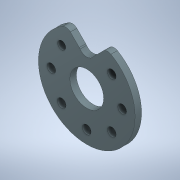
# Autodesk Inventor part: Pulley_middle
Saved by Autodesk Inventor 2020 (Build 240168000, 168)
## iProperties
Created: 2019-10-12
Part Number: Pulley_middle
Material: Generic
Document SubType Name: Modeling
Designer: ayad493
Density: 1 g/cm^3
Appearance: Lead
Author: ayad493
Autodesk Inventor part; units mm, degrees
ref_plane "YZ Plane" through (0, 0, 0) normal (1, 0, 0) x (0, 1, 0)
ref_plane "XZ Plane" through (0, 0, 0) normal (0, 1, 0) x (-1, 0, 0)
ref_plane "XY Plane" through (0, 0, 0) normal (0, 0, 1) x (1, 0, 0)
sketch "Sketch1" plane through (0, 0, 0) normal (0, 0, 1) x (1, 0, 0)
  circle A0 centre (0, 0) radius 18
  dimension "d0" = 36
  constraints: 1 centre point, 1 coincident
  measures "d0" diameter of A0
extrude "Extrusion1" add sketch "Sketch1" along normal blind 2.5
sketch "Sketch2" plane through (0, 0, 2.5) normal (0, 0, 1) x (1, 0, 0)
  line L0 (0, 0) -> (0, 11)
  circle A0 centre (0, 11) radius 1.25
  circle A1 centre (0, 0) radius 5
  circle A2 centre (7.7782, 7.7782) radius 1.25
  circle A3 centre (11, 0) radius 1.25
  circle A4 centre (7.7782, -7.7782) radius 1.25
  circle A5 centre (0, -11) radius 1.25
  circle A6 centre (-7.7782, -7.7782) radius 1.25
  circle A7 centre (-11, 0) radius 1.25
  circle A8 centre (-7.7782, 7.7782) radius 1.25
  dimension "d3" = 11
  dimension "d4" = 2.5
  dimension "d5" = 10
  dimension "d8" = 360
  constraints: 9 centre point, 2 coincident, 2 end point, 1 vertical, 17 other
  measures "d3" distance of L0.start L0.end
  measures "d4" diameter of A0
  measures "d5" diameter of A1
extrude "Extrusion2" cut sketch "Sketch2" against normal through all
sketch "Sketch3" plane through (0, 0, 2.5) normal (0, 0, 1) x (1, 0, 0)
  circle A0 centre (0, 0) radius 15
  circle A1 centre (0, 0) radius 18
  dimension "d12" = 30
  constraints: 2 centre point, 2 coincident
  measures "d12" diameter of A0
extrude "Extrusion3" cut sketch "Sketch3" against normal through all
sketch "Sketch4" plane through (0, 0, 2.5) normal (0, 0, 1) x (1, 0, 0)
  circle A0 centre (0, 11) radius 1.25 projected
  arc A1 (-2.1651, 9.75) -> (2.1651, 9.75) centre (0, 11) ccw
  circle A2 centre (-7.7782, 7.7782) radius 1.25 projected
  circle A3 centre (7.7782, 7.7782) radius 1.25 projected
  circle A4 centre (0, 0) radius 5 projected
  line L0 (2.1651, 9.75) -> (6.1129, 13.6979)
  circle A5 centre (0, 0) radius 15 projected
  line L1 (2.1651, 9.75) -> (7.7482, 9.75) construction
  line L2 (-2.1651, 9.75) -> (-6.1129, 13.6979)
  line L3 (-2.1651, 9.75) -> (3.4181, 9.75) construction
  arc A6 (6.1129, 13.6979) -> (-6.1129, 13.6979) centre (0, 0) ccw
  dimension "d15" = 5
  dimension "d17" = 45
  dimension "d18" = 135
  constraints: 8 end point, 6 point on circle, 2 centre point, 2 equal length, 2 horizontal, 1 coincident, 1 concentric, 1 point on line
  measures "d15" diameter of A1
  measures "d17" angle of L1 L0
  measures "d18" angle of L3 L2
extrude "Extrusion4" cut sketch "Sketch4" against normal blind 10 contours L2 A5 L0 A1 picked at (3.4839, 13.2226)
fillet "Fillet1" radius 2 4 edges at (-6.1129, 13.6979, 1.25) (6.1129, 13.6979, 1.25) (-2.1651, 9.75, 1.25) (2.1651, 9.75, 1.25)
sketch "Sketch5" plane through (0, 0, 2.5) normal (0, 0, 1) x (1, 0, 0)
  line L0 (0, 0) -> (1, 0)
  line L1 (1, 0) -> (1, 1)
  line L2 (1, 1) -> (0, 1)
  line L3 (0, 1) -> (0, 0)
  dimension "d22" = 1
  dimension "d23" = 1
  constraints: 8 end point, 2 parallel, 1 horizontal, 1 perpendicular
  measures "d22" distance of L2.end L1.end
  measures "d23" distance of L1.end L0.end
extrude "Extrusion5" add sketch "Sketch5" along normal blind 1
sketch "Sketch6" plane through (0, 1, 2.5) normal (0, 1, 0) x (1, 0, 0)
  line L0 (2.0766, 0) -> (-2.0766, 0) projected
  line L1 (-15, 2.5) -> (-15, 0) projected
  line L2 (0, 0) -> (-15, 0)
  line L3 (-15, 0) -> (-15, 0.5)
  line L4 (-15, 0.5) -> (0, 0.5)
  line L5 (0, 0.5) -> (0, 0)
  line L6 (0, 0) -> (15, 0)
  line L7 (15, 0) -> (15, 0.5)
  line L8 (15, 0.5) -> (0, 0.5)
  line L9 (0, 0.5) -> (0, 0)
  point P0 (0, 2.5)
  point P1 (0, 0.5)
  dimension "d26" = 0.5
  dimension "d27" = 15
  constraints: 16 end point, 4 parallel, 2 horizontal, 2 perpendicular, 1 midpoint, 1 point on line
  measures "d26" distance of L2.end L3.end
  measures "d27" distance of L8.end L7.end
extrude "Extrusion6" cut sketch "Sketch6" along normal through all both and the other way through all
sketch "Sketch7" plane through (0, 0, 3.5) normal (0, 0, 1) x (1, 0, 0)
  line L0 (1, 1) -> (0, 1) projected
  line L1 (0, 0) -> (1, 0) projected
  line L2 (0, 1) -> (1, 1)
  line L3 (1, 1) -> (1, 0)
  line L4 (1, 0) -> (0, 0)
  line L5 (0, 0) -> (0, 1)
  constraints: 8 end point, 2 parallel, 1 horizontal, 1 perpendicular
extrude "Extrusion7" cut sketch "Sketch7" against normal blind 1
sketch "Sketch8" plane through (0, 0, 2) normal (0, 0, 1) x (1, 0, 0)
  circle A0 centre (0, 0) radius 5.25
  dimension "d32" = 10.5
  constraints: 1 centre point, 1 coincident
  measures "d32" diameter of A0
extrude "Extrusion8" cut sketch "Sketch8" against normal through all
sketch "Sketch9" plane through (0, 0, 0) normal (0, 0, -1) x (-1, 0, 0)
  circle A0 centre (0, -11) radius 1.25 projected
  circle A1 centre (0, -11) radius 1.35
  circle A2 centre (-7.7782, -7.7782) radius 1.25 projected
  circle A3 centre (-7.7782, -7.7782) radius 1.35
  circle A4 centre (-11, 0) radius 1.25 projected
  circle A5 centre (-11, 0) radius 1.35
  circle A6 centre (-7.7782, 7.7782) radius 1.25 projected
  circle A7 centre (-7.7782, 7.7782) radius 1.35
  circle A8 centre (7.7782, -7.7782) radius 1.25 projected
  circle A9 centre (7.7782, -7.7782) radius 1.35
  circle A10 centre (11, 0) radius 1.25 projected
  circle A11 centre (11, 0) radius 1.35
  circle A12 centre (7.7782, 7.7782) radius 1.25 projected
  circle A13 centre (7.7782, 7.7782) radius 1.35
  point P0 (0, 0)
  dimension "d35" = 2.7
  dimension "d36" = 2.7
  dimension "d37" = 2.7
  dimension "d38" = 2.7
  dimension "d39" = 2.7
  dimension "d40" = 2.7
  dimension "d41" = 2.7
  constraints: 7 centre point, 7 coincident
  measures "d35" diameter of A1
  measures "d36" diameter of A3
  measures "d37" diameter of A5
  measures "d38" diameter of A7
  measures "d39" diameter of A9
  measures "d40" diameter of A11
  measures "d41" diameter of A13
extrude "Extrusion9" cut sketch "Sketch9" against normal through all contours A1 | A3 | A5 | A7 | A9 | A10 | A11
body "Solid1"
